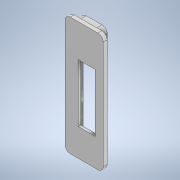
# Autodesk Inventor part: EndSwitchHousing_v02_TopPlate
Saved by Autodesk Inventor 2020 (Build 240168000, 168)
## iProperties
Created: 2020-02-17
Part Number: EndSwitchHousing_v02_TopPlate
Material: Generic
Document SubType Name: Modeling
Designer: Timo
Density: 1 g/cm^3
Appearance: Default
Author: Timo
Autodesk Inventor part; units mm, degrees
ref_plane "YZ Plane" through (0, 0, 0) normal (1, 0, 0) x (0, 1, 0)
ref_plane "XZ Plane" through (0, 0, 0) normal (0, 1, 0) x (-1, 0, 0)
ref_plane "XY Plane" through (0, 0, 0) normal (0, 0, 1) x (1, 0, 0)
sketch "Sketch1" plane through (0, 0, 0) normal (0, 0, 1) x (1, 0, 0)
  line L0 (6.25, -22.5) -> (-8.25, -22.5)
  line L1 (-8.25, -22.5) -> (-8.25, 22.5)
  line L2 (-8.25, 22.5) -> (6.25, 22.5)
  line L3 (6.25, 22.5) -> (6.25, -22.5)
  line L4 (3.25, -12) -> (-3.25, -12)
  line L5 (-3.25, -12) -> (-3.25, 10)
  line L6 (-3.25, 10) -> (3.25, 10)
  line L7 (3.25, 10) -> (3.25, -12)
  line L8 (-11.15, 0) -> (9.15, 0) projected
  line L9 (0, -12) -> (0, 0) construction
  point P0 (6.25, 0)
  dimension "d0" = 6.5
  dimension "d3" = 45
  dimension "d10" = 3
  dimension "d11" = 5
  dimension "d25" = 10
  dimension "d26" = 12
  constraints: 18 end point, 4 parallel, 2 horizontal, 2 midpoint, 2 perpendicular, 1 point on line, 1 vertical
  measures "d0" distance between parallel lines of L7 L5
  measures "d3" distance of L2.end L0.start
  measures "d10" distance between parallel lines of L3 L7
  measures "d11" distance between parallel lines of L1 L5
  measures "d25" distance between parallel lines of L6 L8
  measures "d26" distance between parallel lines of L8 L4
extrude "Extrusion1" add sketch "Sketch1" along normal blind 1.5 contours L0 L1 L8 L5 L4 L7 L3 | L8 L7 L6 L5 L1 L2 L3
fillet "Fillet1" radius 2 4 edges at (6.25, 22.5, 0.75) (-8.25, 22.5, 0.75) (6.25, -22.5, 0.75) (-8.25, -22.5, 0.75)
chamfer "Chamfer1" distance 0.5 angle 45 4 edges at (3.25, -1, 0) (0, 10, 0) (-3.25, -1, 0) (0, -12, 0)
sketch "Sketch2" plane through (0, 0, 0) normal (0, 0, -1) x (-1, 0, 0)
  line L0 (4.65, -21.475) -> (-1.3, -21.475)
  line L1 (-3.3, -19.475) -> (-3.3, 19.475)
  line L2 (-1.3, 21.475) -> (4.65, 21.475)
  line L3 (6.65, 19.475) -> (6.65, -19.475)
  line L4 (3.25, 10) -> (3.25, -12) projected
  arc A0 (-3.3, -19.475) -> (-1.3, -21.475) centre (-1.3, -19.475) ccw
  arc A1 (4.65, -21.475) -> (6.65, -19.475) centre (4.65, -19.475) ccw
  arc A2 (6.65, 19.475) -> (4.65, 21.475) centre (4.65, 19.475) ccw
  arc A3 (-1.3, 21.475) -> (-3.3, 19.475) centre (-1.3, 19.475) ccw
  line L5 (-2.5, 19.475) -> (-2.5, -19.475)
  arc A4 (-2.5, -19.475) -> (-1.3, -20.675) centre (-1.3, -19.475) ccw
  line L6 (-1.3, -20.675) -> (4.65, -20.675)
  arc A5 (4.65, -20.675) -> (5.85, -19.475) centre (4.65, -19.475) ccw
  line L7 (5.85, -19.475) -> (5.85, 19.475)
  arc A6 (5.85, 19.475) -> (4.65, 20.675) centre (4.65, 19.475) ccw
  line L8 (4.65, 20.675) -> (-1.3, 20.675)
  arc A7 (-1.3, 20.675) -> (-2.5, 19.475) centre (-1.3, 19.475) ccw
  line L9 (-2.5, 12) -> (-3.3, 12)
  line L10 (-2.5, -14) -> (-3.3, -14)
  line L11 (3.25, -12) -> (-3.25, -12) projected
  line L12 (-3.25, 10) -> (3.25, 10) projected
  point P0 (0, 0)
  point P1 (-3.3, 21.475)
  point P2 (6.65, 21.475)
  dimension "d12" = 42.95
  dimension "d14" = 9.95
  dimension "d16" = 3.4
  dimension "d17" = 21.475
  dimension "d18" = 2
  dimension "d19" = 0.8
  dimension "d20" = 2
  dimension "d21" = 2
  constraints: 20 end point, 16 point on circle, 8 centre point, 8 point on line, 8 tangent, 4 parallel, 4 perpendicular, 3 equal radius, 1 horizontal, 7 other
  measures "d12" distance between parallel lines of L2 L0
  measures "d14" distance of point (-3.3, 21.475) point (6.65, 21.475)
  measures "d16" distance between parallel lines of L3 L4
  measures "d17" distance from line of point (0, 0) L0
  measures "d18" radius of A0
  measures "d19" distance between parallel lines of L2 L8
  measures "d20" distance between parallel lines of L11 L10
  measures "d21" distance between parallel lines of L12 L9
extrude "Extrusion2" add sketch "Sketch2" along normal blind 3 contours L0 A0 L1 L10 L5 A4 L6 A5 L7 A6 L8 A7 L9 A3 L2 A2 L3 A1
fillet "Fillet2" radius 0.4 4 edges at (3.3, -14, -1.5) (2.5, -14, -1.5) (3.3, 12, -1.5) (2.5, 12, -1.5)
equation "\"d17\" = 0.5 * d12"
equation "\"d21\" = d20"
body "Solid1"
